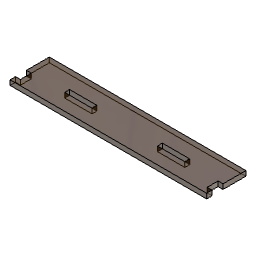
Cap Plate (Autodesk Fusion 360 design; units mm, degrees)
Autodesk Fusion 360 part; units mm, degrees
sketch "Sketch1" plane through (0, 0, 0) normal (0, 0, 1) x (1, 0, 0)
  line L0 (90, -18) -> (-90, -18)
  line L1 (-90, -18) -> (-90, 18)
  line L2 (-90, 18) -> (90, 18)
  line L3 (90, 18) -> (90, -18)
  line L4 (90, -18) -> (-90, 18) construction
  line L5 (-90, -18) -> (90, 18) construction
  line L6 (90, -13) -> (85.5, -13)
  line L7 (85.5, -13) -> (85.5, -3)
  line L8 (85.5, -3) -> (90, -3)
  line L9 (90, -3) -> (90, -13)
  line L10 (-90, -13) -> (-85.5, -13)
  line L11 (-85.5, -13) -> (-85.5, -3)
  line L12 (-85.5, -3) -> (-90, -3)
  line L13 (-90, -3) -> (-90, -13)
  line L14 (-98.0215, -0.75) -> (96.9785, -0.75) construction
  line L15 (55, -3) -> (30, -3)
  line L16 (30, -3) -> (30, 1.5)
  line L17 (30, 1.5) -> (55, 1.5)
  line L18 (55, 1.5) -> (55, -3)
  line L19 (55, -3) -> (30, 1.5) construction
  line L20 (30, -3) -> (55, 1.5) construction
  line L21 (-30, -3) -> (-55, -3)
  line L22 (-55, -3) -> (-55, 1.5)
  line L23 (-55, 1.5) -> (-30, 1.5)
  line L24 (-30, 1.5) -> (-30, -3)
  line L25 (-30, -3) -> (-55, 1.5) construction
  line L26 (-55, -3) -> (-30, 1.5) construction
  point P0 (42.5, -0.75)
  point P1 (-42.5, -0.75)
  dimension "d1" = 180
  dimension "d2" = 36
  dimension "d3" = 4.5
  dimension "d4" = 10
  dimension "d5" = 4.5
  dimension "d6" = 10
  dimension "d7" = 5
  dimension "d8" = 5
  dimension "d9" = 17.25
  dimension "d10" = 25
  dimension "d11" = 4.5
  dimension "d12" = 25
  dimension "d13" = 4.5
  dimension "d14" = 35
  dimension "d15" = 35
  constraint horizontal L0
  constraint perpendicular L0 L1
  constraint parallel L0 L2
  constraint parallel L1 L3
  constraint coincident L4 origin
  constraint coincident L5 origin
  constraint horizontal L6
  constraint vertical L7
  constraint horizontal L8
  constraint vertical L9
  constraint coincident L3 L6.start
  constraint horizontal L10
  constraint vertical L11
  constraint horizontal L12
  constraint vertical L13
  constraint coincident L1 L10.start
  constraint perpendicular L1 L14
  constraint horizontal L15
  constraint perpendicular L15 L16
  constraint parallel L15 L17
  constraint parallel L16 L18
  constraint coincident L19 P0
  constraint coincident L20 P0
  constraint coincident L14 P0
  constraint horizontal L21
  constraint perpendicular L21 L22
  constraint parallel L21 L23
  constraint parallel L22 L24
  constraint coincident L25 P1
  constraint coincident L26 P1
  constraint coincident L14 P1
  measures "d1" distance of L1.end L2.end
  measures "d2" distance of L0.end L1.end
  measures "d3" distance of L6.start L6.end
  measures "d4" distance of L6.start L8.end
  measures "d5" distance of L10.start L10.end
  measures "d6" distance of L10.start L12.end
  measures "d7" distance of L0 L6
  measures "d8" distance of L0 L10
  measures "d9" distance of L0 L14
  measures "d10" distance of L16.end L17.end
  measures "d11" distance of L15.end L16.end
  measures "d12" distance of L22.end L23.end
  measures "d13" distance of L21.end L22.end
  measures "d14" distance of L1 L22
  measures "d15" distance of L3 L18
extrude "Extrude1" add sketch "Sketch1" along normal blind 4.5 contours L0 L1 L2 L3 L6 L7 L8 L10 L11 L12
